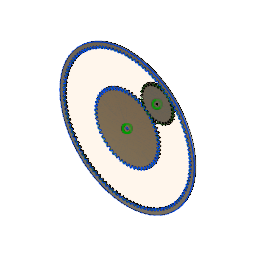
cncgearv3 (Autodesk Fusion 360 design; units mm, degrees)
description: Spur Gear; Module: 5.000000; Num Teeth: 56; Pressure Angle: 20.000000;
description: Spur Gear; Module: 5.000000; Num Teeth: 28; Pressure Angle: 20.000000;
description: Internal Gear; Module: 5.000000; Num Teeth: 112; Pressure Angle: 20.000000;
Autodesk Fusion 360 part; units mm, degrees
(part 1 of 4)
sketch "sketch 243" plane through (0, 0, 0) normal (0, 1, 0) x (1, 0, 0)
  spline S0 degree 3 poles (-118.3417, 63.013) (-119.0377, 63.2246) (-119.8918, 63.4524) (-120.912, 63.6705) knots 0 0 0 0 1 1 1 1
  arc A0 (-129.7827, 64.6689) -> (-131.4784, 61.1478) centre (0, 0) ccw
  spline S1 degree 3 poles (-125.167, 54.8349) (-124.3604, 54.1733) (-123.6498, 53.6475) (-123.0504, 53.2353) knots 0 0 0 0 1 1 1 1
  spline S2 degree 3 poles (-137.4981, 46.0424) (-134.792, 43.4861) (-132.4072, 41.6981) (-130.5195, 40.4758) knots 0 0 0 0 1 1 1 1
  spline S3 degree 3 poles (-130.5195, 40.4758) (-129.6439, 39.9087) (-128.8789, 39.4658) (-128.2371, 39.1233) knots 0 0 0 0 1 1 1 1
  spline S4 degree 3 poles (-129.3963, 35.0996) (-130.122, 35.1511) (-131.0054, 35.183) (-132.0485, 35.1687) knots 0 0 0 0 1 1 1 1
  arc A1 (-128.0426, 38.6549) -> (-128.2371, 39.1233) centre (-128.4255, 38.7705) ccw
  arc A2 (-136.2073, 49.7313) -> (-137.4981, 46.0424) centre (0, 0) ccw
  arc A3 (-129.3963, 35.0996) -> (-128.9824, 35.3927) centre (-129.3682, 35.4986) ccw
  spline S5 degree 3 poles (-141.7886, 30.358) (-138.8134, 28.1207) (-136.2434, 26.611) (-134.2307, 25.6078) knots 0 0 0 0 1 1 1 1
  arc A4 (-132.5126, 20.3911) -> (-132.1341, 20.7287) centre (-132.5293, 20.7907) ccw
  spline S6 degree 3 poles (-135.1558, 20.1628) (-137.3869, 19.8806) (-140.3113, 19.3045) (-143.8585, 18.1754) knots 0 0 0 0 1 1 1 1
  arc A5 (-133.4338, 9.1936) -> (-133.6242, 5.8041) centre (0, 0) ccw
  spline S7 degree 3 poles (-144.2961, 14.2918) (-141.0891, 12.4017) (-138.3662, 11.1893) (-136.2538, 10.4177) knots 0 0 0 0 1 1 1 1
  arc A6 (-116.2308, 66.1779) -> (-116.3162, 66.6779) centre (-116.5784, 66.3758) ccw
  arc A7 (-118.3417, 63.013) -> (-117.8729, 63.2067) centre (-118.2255, 63.3957) ccw
  arc A8 (-144.989, 1.9541) -> (-144.989, -1.9541) centre (0, 0) ccw
  spline S8 degree 3 poles (-144.989, -1.9541) (-141.5905, -3.4732) (-138.749, -4.3732) (-136.5635, -4.9034) knots 0 0 0 0 1 1 1 1
  spline S9 degree 3 poles (-136.5635, 4.9034) (-138.749, 4.3732) (-141.5905, 3.4732) (-144.989, 1.9541) knots 0 0 0 0 1 1 1 1
  arc A9 (-133.4338, 9.1936) -> (-133.7277, 9.607) centre (-133.8329, 9.2211) ccw
  arc A10 (-122.9095, 52.7481) -> (-124.2087, 49.6116) centre (0, 0) ccw
  spline S10 degree 3 poles (-110.5424, 75.8668) (-111.2103, 76.1551) (-112.0336, 76.477) (-113.0228, 76.808) knots 0 0 0 0 1 1 1 1
  spline S11 degree 3 poles (-118.2404, 68.5043) (-117.5129, 67.7566) (-116.8657, 67.1545) (-116.3162, 66.6779) knots 0 0 0 0 1 1 1 1
  spline S12 degree 3 poles (-120.912, 63.6705) (-123.1111, 64.141) (-126.0616, 64.5631) (-129.7827, 64.6689) knots 0 0 0 0 1 1 1 1
  arc A11 (-122.9095, 52.7481) -> (-123.0504, 53.2353) centre (-123.2771, 52.9058) ccw
  spline S13 degree 3 poles (-127.2805, 49.7323) (-129.5185, 49.9537) (-132.4978, 50.0427) (-136.2073, 49.7313) knots 0 0 0 0 1 1 1 1
  arc A12 (-128.0426, 38.6549) -> (-128.9824, 35.3927) centre (0, 0) ccw
  spline S14 degree 3 poles (-131.4784, 61.1478) (-129.0756, 58.3046) (-126.906, 56.2608) (-125.167, 54.8349) knots 0 0 0 0 1 1 1 1
  arc A13 (-140.919, 34.1682) -> (-141.7886, 30.358) centre (0, 0) ccw
  arc A14 (-131.5655, 24.0756) -> (-131.8112, 24.5193) centre (-131.9589, 24.1476) ccw
  spline S15 degree 3 poles (-134.2307, 25.6078) (-133.2971, 25.1423) (-132.4873, 24.7878) (-131.8112, 24.5193) knots 0 0 0 0 1 1 1 1
  arc A15 (-131.5655, 24.0756) -> (-132.1341, 20.7287) centre (0, 0) ccw
  spline S16 degree 3 poles (-132.5126, 20.3911) (-133.2394, 20.361) (-134.1209, 20.2939) (-135.1558, 20.1628) knots 0 0 0 0 1 1 1 1
  arc A16 (-143.8585, 18.1754) -> (-144.2961, 14.2918) centre (0, 0) ccw
  arc A17 (-124.6528, 49.3667) -> (-124.2087, 49.6116) centre (-124.5801, 49.76) ccw
  arc A18 (-116.2308, 66.1779) -> (-117.8729, 63.2067) centre (0, 0) ccw
  spline S17 degree 3 poles (-132.0485, 35.1687) (-134.2971, 35.1381) (-137.2676, 34.893) (-140.919, 34.1682) knots 0 0 0 0 1 1 1 1
  spline S18 degree 3 poles (-136.2538, 10.4177) (-135.274, 10.0596) (-134.4296, 9.798) (-133.7277, 9.607) knots 0 0 0 0 1 1 1 1
  spline S19 degree 3 poles (-133.9625, 5.4262) (-134.6814, 5.3149) (-135.5497, 5.1495) (-136.5635, 4.9034) knots 0 0 0 0 1 1 1 1
  arc A19 (-133.7277, -9.607) -> (-133.4338, -9.1936) centre (-133.8329, -9.2211) ccw
  arc A20 (-133.6242, -5.8041) -> (-133.9625, -5.4262) centre (-134.0238, -5.8214) ccw
  arc A21 (-133.6242, -5.8041) -> (-133.4338, -9.1936) centre (0, 0) ccw
  spline S20 degree 3 poles (-123.8053, 75.4842) (-121.7359, 72.3898) (-119.8088, 70.116) (-118.2404, 68.5043) knots 0 0 0 0 1 1 1 1
  spline S21 degree 3 poles (-124.6528, 49.3667) (-125.3681, 49.4991) (-126.2424, 49.6298) (-127.2805, 49.7323) knots 0 0 0 0 1 1 1 1
  arc A22 (-133.9625, 5.4262) -> (-133.6242, 5.8041) centre (-134.0238, 5.8214) ccw
  arc A23 (-121.726, 78.7934) -> (-123.8053, 75.4842) centre (0, 0) ccw
  spline S22 degree 3 poles (-113.0228, 76.808) (-115.1555, 77.5218) (-118.0402, 78.2715) (-121.726, 78.7934) knots 0 0 0 0 1 1 1 1
  spline S23 degree 3 poles (-136.2538, -10.4177) (-138.3662, -11.1893) (-141.0891, -12.4017) (-144.2961, -14.2918) knots 0 0 0 0 1 1 1 1
  spline S24 degree 3 poles (-135.1558, -20.1628) (-134.1209, -20.2939) (-133.2394, -20.361) (-132.5126, -20.3911) knots 0 0 0 0 1 1 1 1
  spline S25 degree 3 poles (-134.2307, -25.6078) (-136.2434, -26.611) (-138.8134, -28.1207) (-141.7886, -30.358) knots 0 0 0 0 1 1 1 1
  spline S26 degree 3 poles (-128.2371, -39.1233) (-128.8789, -39.4658) (-129.6439, -39.9087) (-130.5195, -40.4758) knots 0 0 0 0 1 1 1 1
  arc A24 (-110.0549, -76.0068) -> (-110.5424, -75.8668) centre (-110.384, -76.2341) ccw
  arc A25 (-128.2371, -39.1233) -> (-128.0426, -38.6549) centre (-128.4255, -38.7705) ccw
  spline S27 degree 3 poles (-108.1193, -79.2819) (-108.6119, -79.8171) (-109.1877, -80.4878) (-109.8269, -81.3123) knots 0 0 0 0 1 1 1 1
  arc A26 (-110.0549, -76.0068) -> (-108.0904, -78.7755) centre (0, 0) ccw
  arc A27 (-128.9824, -35.3927) -> (-129.3963, -35.0996) centre (-129.3682, -35.4986) ccw
  spline S28 degree 3 poles (-136.2073, -49.7313) (-132.4978, -50.0427) (-129.5185, -49.9537) (-127.2805, -49.7323) knots 0 0 0 0 1 1 1 1
  spline S29 degree 3 poles (-103.7124, -88.9796) (-102.7664, -88.5399) (-101.9843, -88.1278) (-101.3529, -87.7666) knots 0 0 0 0 1 1 1 1
  spline S30 degree 3 poles (-109.8269, -81.3123) (-111.205, -83.0895) (-112.8654, -85.5648) (-114.5753, -88.8714) knots 0 0 0 0 1 1 1 1
  spline S31 degree 3 poles (-118.2404, -68.5043) (-119.8088, -70.116) (-121.7359, -72.3898) (-123.8053, -75.4842) knots 0 0 0 0 1 1 1 1
  spline S32 degree 3 poles (-112.1386, -91.9269) (-108.5344, -90.9957) (-105.7517, -89.9277) (-103.7124, -88.9796) knots 0 0 0 0 1 1 1 1
  arc A28 (-114.5753, -88.8714) -> (-112.1386, -91.9269) centre (0, 0) ccw
  spline S33 degree 3 poles (-129.7827, -64.6689) (-126.0616, -64.5631) (-123.1111, -64.141) (-120.912, -63.6705) knots 0 0 0 0 1 1 1 1
  arc A29 (-100.8528, -87.8511) -> (-101.3529, -87.7666) centre (-101.1544, -88.1139) ccw
  arc A30 (-132.1341, -20.7287) -> (-131.5655, -24.0756) centre (0, 0) ccw
  arc A31 (-131.8112, -24.5193) -> (-131.5655, -24.0756) centre (-131.9589, -24.1476) ccw
  arc A32 (-123.0504, -53.2353) -> (-122.9095, -52.7481) centre (-123.2771, -52.9058) ccw
  spline S34 degree 3 poles (-125.167, -54.8349) (-126.906, -56.2608) (-129.0756, -58.3046) (-131.4784, -61.1478) knots 0 0 0 0 1 1 1 1
  arc A33 (-131.4784, -61.1478) -> (-129.7827, -64.6689) centre (0, 0) ccw
  arc A34 (-116.3162, -66.6779) -> (-116.2308, -66.1779) centre (-116.5784, -66.3758) ccw
  spline S35 degree 3 poles (-136.5635, -4.9034) (-135.5497, -5.1495) (-134.6814, -5.3149) (-133.9625, -5.4262) knots 0 0 0 0 1 1 1 1
  spline S36 degree 3 poles (-130.5195, -40.4758) (-132.4072, -41.6981) (-134.792, -43.4861) (-137.4981, -46.0424) knots 0 0 0 0 1 1 1 1
  arc A35 (-117.8729, -63.2067) -> (-118.3417, -63.013) centre (-118.2255, -63.3957) ccw
  arc A36 (-128.9824, -35.3927) -> (-128.0426, -38.6549) centre (0, 0) ccw
  spline S37 degree 3 poles (-116.3162, -66.6779) (-116.8657, -67.1545) (-117.5129, -67.7566) (-118.2404, -68.5043) knots 0 0 0 0 1 1 1 1
  arc A37 (-117.8729, -63.2067) -> (-116.2308, -66.1779) centre (0, 0) ccw
  spline S38 degree 3 poles (-131.8112, -24.5193) (-132.4873, -24.7878) (-133.2971, -25.1423) (-134.2307, -25.6078) knots 0 0 0 0 1 1 1 1
  arc A38 (-137.4981, -46.0424) -> (-136.2073, -49.7313) centre (0, 0) ccw
  spline S39 degree 3 poles (-132.0485, -35.1687) (-131.0054, -35.183) (-130.122, -35.1511) (-129.3963, -35.0996) knots 0 0 0 0 1 1 1 1
  spline S40 degree 3 poles (-143.8585, -18.1754) (-140.3113, -19.3045) (-137.3869, -19.8806) (-135.1558, -20.1628) knots 0 0 0 0 1 1 1 1
  spline S41 degree 3 poles (-140.919, -34.1682) (-137.2676, -34.893) (-134.2971, -35.1381) (-132.0485, -35.1687) knots 0 0 0 0 1 1 1 1
  arc A39 (-141.7886, -30.358) -> (-140.919, -34.1682) centre (0, 0) ccw
  arc A40 (-124.2087, -49.6116) -> (-122.9095, -52.7481) centre (0, 0) ccw
  arc A41 (-124.2087, -49.6116) -> (-124.6528, -49.3667) centre (-124.5801, -49.76) ccw
  spline S42 degree 3 poles (-123.0504, -53.2353) (-123.6498, -53.6475) (-124.3604, -54.1733) (-125.167, -54.8349) knots 0 0 0 0 1 1 1 1
  spline S43 degree 3 poles (-120.912, -63.6705) (-119.8918, -63.4524) (-119.0377, -63.2246) (-118.3417, -63.013) knots 0 0 0 0 1 1 1 1
  spline S44 degree 3 poles (-121.726, -78.7934) (-118.0402, -78.2715) (-115.1555, -77.5218) (-113.0228, -76.808) knots 0 0 0 0 1 1 1 1
  arc A42 (-123.8053, -75.4842) -> (-121.726, -78.7934) centre (0, 0) ccw
  spline S45 degree 3 poles (-113.0228, -76.808) (-112.0336, -76.477) (-111.2103, -76.1551) (-110.5424, -75.8668) knots 0 0 0 0 1 1 1 1
  arc A43 (-144.2961, -14.2918) -> (-143.8585, -18.1754) centre (0, 0) ccw
  spline S46 degree 3 poles (-127.2805, -49.7323) (-126.2424, -49.6298) (-125.3681, -49.4991) (-124.6528, -49.3667) knots 0 0 0 0 1 1 1 1
  arc A44 (-108.1193, -79.2819) -> (-108.0904, -78.7755) centre (-108.4136, -79.0111) ccw
  arc A45 (-132.1341, -20.7287) -> (-132.5126, -20.3911) centre (-132.5293, -20.7907) ccw
  spline S47 degree 3 poles (-133.7277, -9.607) (-134.4296, -9.798) (-135.274, -10.0596) (-136.2538, -10.4177) knots 0 0 0 0 1 1 1 1
  spline S48 degree 3 poles (-75.8668, -110.5424) (-76.1551, -111.2103) (-76.477, -112.0336) (-76.808, -113.0228) knots 0 0 0 0 1 1 1 1
  spline S49 degree 3 poles (-93.0977, -100.0322) (-92.2069, -99.4894) (-91.4759, -98.9923) (-90.8889, -98.5627) knots 0 0 0 0 1 1 1 1
  spline S50 degree 3 poles (-87.7666, -101.3529) (-88.1278, -101.9843) (-88.5399, -102.7664) (-88.9796, -103.7124) knots 0 0 0 0 1 1 1 1
  arc A46 (-78.7755, -108.0904) -> (-79.2819, -108.1193) centre (-79.0111, -108.4136) ccw
  arc A47 (-75.8668, -110.5424) -> (-76.0068, -110.0549) centre (-76.2341, -110.384) ccw
  spline S51 degree 3 poles (-76.808, -113.0228) (-77.5218, -115.1555) (-78.2715, -118.0402) (-78.7934, -121.726) knots 0 0 0 0 1 1 1 1
  arc A48 (-90.3825, -98.5907) -> (-90.8889, -98.5627) centre (-90.6528, -98.8855) ccw
  arc A49 (-78.7934, -121.726) -> (-75.4842, -123.8053) centre (0, 0) ccw
  spline S52 degree 3 poles (-75.4842, -123.8053) (-72.3898, -121.7359) (-70.116, -119.8088) (-68.5043, -118.2404) knots 0 0 0 0 1 1 1 1
  arc A50 (-66.1779, -116.2308) -> (-63.2067, -117.8729) centre (0, 0) ccw
  arc A51 (-63.013, -118.3417) -> (-63.2067, -117.8729) centre (-63.3957, -118.2255) ccw
  spline S53 degree 3 poles (-100.0322, -93.0977) (-101.2027, -95.018) (-102.5755, -97.6637) (-103.9044, -101.1409) knots 0 0 0 0 1 1 1 1
  spline S54 degree 3 poles (-88.9796, -103.7124) (-89.9277, -105.7517) (-90.9957, -108.5344) (-91.9269, -112.1386) knots 0 0 0 0 1 1 1 1
  arc A52 (-100.8528, -87.8511) -> (-98.5907, -90.3825) centre (0, 0) ccw
  spline S55 degree 3 poles (-81.3123, -109.8269) (-80.4878, -109.1877) (-79.8171, -108.6119) (-79.2819, -108.1193) knots 0 0 0 0 1 1 1 1
  spline S56 degree 3 poles (-88.8714, -114.5753) (-85.5648, -112.8654) (-83.0895, -111.205) (-81.3123, -109.8269) knots 0 0 0 0 1 1 1 1
  arc A53 (-91.9269, -112.1386) -> (-88.8714, -114.5753) centre (0, 0) ccw
  arc A54 (-90.3825, -98.5907) -> (-87.8511, -100.8528) centre (0, 0) ccw
  arc A55 (-66.1779, -116.2308) -> (-66.6779, -116.3162) centre (-66.3758, -116.5784) ccw
  spline S57 degree 3 poles (-101.1409, -103.9044) (-97.6637, -102.5755) (-95.018, -101.2027) (-93.0977, -100.0322) knots 0 0 0 0 1 1 1 1
  arc A56 (-78.7755, -108.0904) -> (-76.0068, -110.0549) centre (0, 0) ccw
  spline S58 degree 3 poles (-68.5043, -118.2404) (-67.7566, -117.5129) (-67.1545, -116.8657) (-66.6779, -116.3162) knots 0 0 0 0 1 1 1 1
  arc A57 (-103.9044, -101.1409) -> (-101.1409, -103.9044) centre (0, 0) ccw
  spline S59 degree 3 poles (-63.013, -118.3417) (-63.2246, -119.0377) (-63.4524, -119.8918) (-63.6705, -120.912) knots 0 0 0 0 1 1 1 1
  arc A58 (-87.7666, -101.3529) -> (-87.8511, -100.8528) centre (-88.1139, -101.1544) ccw
  spline S60 degree 3 poles (-54.8349, -125.167) (-54.1733, -124.3604) (-53.6475, -123.6498) (-53.2353, -123.0504) knots 0 0 0 0 1 1 1 1
  spline S61 degree 3 poles (-98.5627, -90.8889) (-98.9923, -91.4759) (-99.4894, -92.2069) (-100.0322, -93.0977) knots 0 0 0 0 1 1 1 1
  arc A59 (-98.5627, -90.8889) -> (-98.5907, -90.3825) centre (-98.8855, -90.6528) ccw
  spline S62 degree 3 poles (-63.6705, -120.912) (-64.141, -123.1111) (-64.5631, -126.0616) (-64.6689, -129.7827) knots 0 0 0 0 1 1 1 1
  spline S63 degree 3 poles (-61.1478, -131.4784) (-58.3046, -129.0756) (-56.2608, -126.906) (-54.8349, -125.167) knots 0 0 0 0 1 1 1 1
  arc A60 (-88.8714, 114.5753) -> (-91.9269, 112.1386) centre (0, 0) ccw
  spline S64 degree 3 poles (-88.9796, 103.7124) (-88.5399, 102.7664) (-88.1278, 101.9843) (-87.7666, 101.3529) knots 0 0 0 0 1 1 1 1
  arc A61 (-87.8511, 100.8528) -> (-87.7666, 101.3529) centre (-88.1139, 101.1544) ccw
  spline S65 degree 3 poles (-90.8889, 98.5627) (-91.4759, 98.9923) (-92.2069, 99.4894) (-93.0977, 100.0322) knots 0 0 0 0 1 1 1 1
  arc A62 (-90.8889, 98.5627) -> (-90.3825, 98.5907) centre (-90.6528, 98.8855) ccw
  spline S66 degree 3 poles (-93.0977, 100.0322) (-95.018, 101.2027) (-97.6637, 102.5755) (-101.1409, 103.9044) knots 0 0 0 0 1 1 1 1
  arc A63 (-64.6689, -129.7827) -> (-61.1478, -131.4784) centre (0, 0) ccw
  spline S67 degree 3 poles (-91.9269, 112.1386) (-90.9957, 108.5344) (-89.9277, 105.7517) (-88.9796, 103.7124) knots 0 0 0 0 1 1 1 1
  spline S68 degree 3 poles (-103.9044, 101.1409) (-102.5755, 97.6637) (-101.2027, 95.018) (-100.0322, 93.0977) knots 0 0 0 0 1 1 1 1
  spline S69 degree 3 poles (-81.3123, 109.8269) (-83.0895, 111.205) (-85.5648, 112.8654) (-88.8714, 114.5753) knots 0 0 0 0 1 1 1 1
  arc A64 (-87.8511, 100.8528) -> (-90.3825, 98.5907) centre (0, 0) ccw
  arc A65 (-98.5907, 90.3825) -> (-100.8528, 87.8511) centre (0, 0) ccw
  arc A66 (-108.0904, 78.7755) -> (-108.1193, 79.2819) centre (-108.4136, 79.0111) ccw
  arc A67 (-110.5424, 75.8668) -> (-110.0549, 76.0068) centre (-110.384, 76.2341) ccw
  arc A68 (-108.0904, 78.7755) -> (-110.0549, 76.0068) centre (0, 0) ccw
  arc A69 (24.5193, -131.8112) -> (24.0756, -131.5655) centre (24.1476, -131.9589) ccw
  arc A70 (14.2918, -144.2961) -> (18.1754, -143.8585) centre (0, 0) ccw
  spline S70 degree 3 poles (20.1628, -135.1558) (20.2939, -134.1209) (20.361, -133.2394) (20.3911, -132.5126) knots 0 0 0 0 1 1 1 1
  spline S71 degree 3 poles (18.1754, -143.8585) (19.3045, -140.3113) (19.8806, -137.3869) (20.1628, -135.1558) knots 0 0 0 0 1 1 1 1
  arc A71 (20.7287, -132.1341) -> (20.3911, -132.5126) centre (20.7907, -132.5293) ccw
  spline S72 degree 3 poles (25.6078, -134.2307) (26.611, -136.2434) (28.1207, -138.8134) (30.358, -141.7886) knots 0 0 0 0 1 1 1 1
  spline S73 degree 3 poles (34.1682, -140.919) (34.893, -137.2676) (35.1381, -134.2971) (35.1687, -132.0485) knots 0 0 0 0 1 1 1 1
  arc A72 (35.3927, -128.9824) -> (35.0996, -129.3963) centre (35.4986, -129.3682) ccw
  arc A73 (35.3927, -128.9824) -> (38.6549, -128.0426) centre (0, 0) ccw
  spline S74 degree 3 poles (-103.7124, 88.9796) (-105.7517, 89.9277) (-108.5344, 90.9957) (-112.1386, 91.9269) knots 0 0 0 0 1 1 1 1
  spline S75 degree 3 poles (-100.0322, 93.0977) (-99.4894, 92.2069) (-98.9923, 91.4759) (-98.5627, 90.8889) knots 0 0 0 0 1 1 1 1
  spline S76 degree 3 poles (-109.8269, 81.3123) (-109.1877, 80.4878) (-108.6119, 79.8171) (-108.1193, 79.2819) knots 0 0 0 0 1 1 1 1
  spline S77 degree 3 poles (40.4758, -130.5195) (41.6981, -132.4072) (43.4861, -134.792) (46.0424, -137.4981) knots 0 0 0 0 1 1 1 1
  spline S78 degree 3 poles (39.1233, -128.2371) (39.4658, -128.8789) (39.9087, -129.6439) (40.4758, -130.5195) knots 0 0 0 0 1 1 1 1
  arc A74 (53.2353, -123.0504) -> (52.7481, -122.9095) centre (52.9058, -123.2771) ccw
  arc A75 (49.6116, -124.2087) -> (49.3667, -124.6528) centre (49.76, -124.5801) ccw
  spline S79 degree 3 poles (-114.5753, 88.8714) (-112.8654, 85.5648) (-111.205, 83.0895) (-109.8269, 81.3123) knots 0 0 0 0 1 1 1 1
  spline S80 degree 3 poles (24.5193, -131.8112) (24.7878, -132.4873) (25.1423, -133.2971) (25.6078, -134.2307) knots 0 0 0 0 1 1 1 1
  spline S81 degree 3 poles (35.1687, -132.0485) (35.183, -131.0054) (35.1511, -130.122) (35.0996, -129.3963) knots 0 0 0 0 1 1 1 1
  arc A76 (-101.3529, 87.7666) -> (-100.8528, 87.8511) centre (-101.1544, 88.1139) ccw
  arc A77 (20.7287, -132.1341) -> (24.0756, -131.5655) centre (0, 0) ccw
  arc A78 (30.358, -141.7886) -> (34.1682, -140.919) centre (0, 0) ccw
  arc A79 (39.1233, -128.2371) -> (38.6549, -128.0426) centre (38.7705, -128.4255) ccw
  arc A80 (46.0424, -137.4981) -> (49.7313, -136.2073) centre (0, 0) ccw
  spline S82 degree 3 poles (53.2353, -123.0504) (53.6475, -123.6498) (54.1733, -124.3604) (54.8349, -125.167) knots 0 0 0 0 1 1 1 1
  spline S83 degree 3 poles (49.7313, -136.2073) (50.0427, -132.4978) (49.9537, -129.5185) (49.7323, -127.2805) knots 0 0 0 0 1 1 1 1
  arc A81 (-98.5907, 90.3825) -> (-98.5627, 90.8889) centre (-98.8855, 90.6528) ccw
  spline S84 degree 3 poles (-101.3529, 87.7666) (-101.9843, 88.1278) (-102.7664, 88.5399) (-103.7124, 88.9796) knots 0 0 0 0 1 1 1 1
  arc A82 (-112.1386, 91.9269) -> (-114.5753, 88.8714) centre (0, 0) ccw
  arc A83 (-101.1409, 103.9044) -> (-103.9044, 101.1409) centre (0, 0) ccw
  spline S85 degree 3 poles (137.4981, -46.0424) (134.792, -43.4861) (132.4072, -41.6981) (130.5195, -40.4758) knots 0 0 0 0 1 1 1 1
  spline S86 degree 3 poles (90.8889, -98.5627) (91.4759, -98.9923) (92.2069, -99.4894) (93.0977, -100.0322) knots 0 0 0 0 1 1 1 1
  arc A84 (88.8714, -114.5753) -> (91.9269, -112.1386) centre (0, 0) ccw
  arc A85 (128.0426, -38.6549) -> (128.9824, -35.3927) centre (0, 0) ccw
  arc A86 (49.6116, -124.2087) -> (52.7481, -122.9095) centre (0, 0) ccw
  spline S87 degree 3 poles (101.3529, -87.7666) (101.9843, -88.1278) (102.7664, -88.5399) (103.7124, -88.9796) knots 0 0 0 0 1 1 1 1
  arc A87 (108.0904, -78.7755) -> (110.0549, -76.0068) centre (0, 0) ccw
  arc A88 (116.2308, -66.1779) -> (116.3162, -66.6779) centre (116.5784, -66.3758) ccw
  spline S88 degree 3 poles (88.9796, -103.7124) (88.5399, -102.7664) (88.1278, -101.9843) (87.7666, -101.3529) knots 0 0 0 0 1 1 1 1
  arc A89 (110.5424, -75.8668) -> (110.0549, -76.0068) centre (110.384, -76.2341) ccw
  arc A90 (63.2067, -117.8729) -> (66.1779, -116.2308) centre (0, 0) ccw
  spline S89 degree 3 poles (103.9044, -101.1409) (102.5755, -97.6637) (101.2027, -95.018) (100.0322, -93.0977) knots 0 0 0 0 1 1 1 1
  spline S90 degree 3 poles (66.6779, -116.3162) (67.1545, -116.8657) (67.7566, -117.5129) (68.5043, -118.2404) knots 0 0 0 0 1 1 1 1
  arc A91 (122.9095, -52.7481) -> (123.0504, -53.2353) centre (123.2771, -52.9058) ccw
  spline S91 degree 3 poles (78.7934, -121.726) (78.2715, -118.0402) (77.5218, -115.1555) (76.808, -113.0228) knots 0 0 0 0 1 1 1 1
  arc A92 (112.1386, -91.9269) -> (114.5753, -88.8714) centre (0, 0) ccw
  arc A93 (121.726, -78.7934) -> (123.8053, -75.4842) centre (0, 0) ccw
  spline S92 degree 3 poles (76.808, -113.0228) (76.477, -112.0336) (76.1551, -111.2103) (75.8668, -110.5424) knots 0 0 0 0 1 1 1 1
  arc A94 (75.4842, -123.8053) -> (78.7934, -121.726) centre (0, 0) ccw
  arc A95 (61.1478, -131.4784) -> (64.6689, -129.7827) centre (0, 0) ccw
  spline S93 degree 3 poles (68.5043, -118.2404) (70.116, -119.8088) (72.3898, -121.7359) (75.4842, -123.8053) knots 0 0 0 0 1 1 1 1
  arc A96 (87.8511, -100.8528) -> (87.7666, -101.3529) centre (88.1139, -101.1544) ccw
  arc A97 (76.0068, -110.0549) -> (75.8668, -110.5424) centre (76.2341, -110.384) ccw
  spline S94 degree 3 poles (110.5424, -75.8668) (111.2103, -76.1551) (112.0336, -76.477) (113.0228, -76.808) knots 0 0 0 0 1 1 1 1
  spline S95 degree 3 poles (100.0322, -93.0977) (99.4894, -92.2069) (98.9923, -91.4759) (98.5627, -90.8889) knots 0 0 0 0 1 1 1 1
  arc A98 (101.3529, -87.7666) -> (100.8528, -87.8511) centre (101.1544, -88.1139) ccw
  arc A99 (101.1409, -103.9044) -> (103.9044, -101.1409) centre (0, 0) ccw
  spline S96 degree 3 poles (109.8269, -81.3123) (109.1877, -80.4878) (108.6119, -79.8171) (108.1193, -79.2819) knots 0 0 0 0 1 1 1 1
  spline S97 degree 3 poles (113.0228, -76.808) (115.1555, -77.5218) (118.0402, -78.2715) (121.726, -78.7934) knots 0 0 0 0 1 1 1 1
  spline S98 degree 3 poles (125.167, -54.8349) (124.3604, -54.1733) (123.6498, -53.6475) (123.0504, -53.2353) knots 0 0 0 0 1 1 1 1
  arc A100 (63.2067, -117.8729) -> (63.013, -118.3417) centre (63.3957, -118.2255) ccw
  arc A101 (122.9095, -52.7481) -> (124.2087, -49.6116) centre (0, 0) ccw
  spline S99 degree 3 poles (131.4784, -61.1478) (129.0756, -58.3046) (126.906, -56.2608) (125.167, -54.8349) knots 0 0 0 0 1 1 1 1
  arc A102 (87.8511, -100.8528) -> (90.3825, -98.5907) centre (0, 0) ccw
  arc A103 (90.8889, -98.5627) -> (90.3825, -98.5907) centre (90.6528, -98.8855) ccw
  spline S100 degree 3 poles (118.2404, -68.5043) (117.5129, -67.7566) (116.8657, -67.1545) (116.3162, -66.6779) knots 0 0 0 0 1 1 1 1
  spline S101 degree 3 poles (91.9269, -112.1386) (90.9957, -108.5344) (89.9277, -105.7517) (88.9796, -103.7124) knots 0 0 0 0 1 1 1 1
  arc A104 (116.2308, -66.1779) -> (117.8729, -63.2067) centre (0, 0) ccw
  spline S102 degree 3 poles (120.912, -63.6705) (123.1111, -64.141) (126.0616, -64.5631) (129.7827, -64.6689) knots 0 0 0 0 1 1 1 1
  spline S103 degree 3 poles (118.3417, -63.013) (119.0377, -63.2246) (119.8918, -63.4524) (120.912, -63.6705) knots 0 0 0 0 1 1 1 1
  arc A105 (98.5907, -90.3825) -> (100.8528, -87.8511) centre (0, 0) ccw
  arc A106 (66.6779, -116.3162) -> (66.1779, -116.2308) centre (66.3758, -116.5784) ccw
  spline S104 degree 3 poles (123.8053, -75.4842) (121.7359, -72.3898) (119.8088, -70.116) (118.2404, -68.5043) knots 0 0 0 0 1 1 1 1
  spline S105 degree 3 poles (93.0977, -100.0322) (95.018, -101.2027) (97.6637, -102.5755) (101.1409, -103.9044) knots 0 0 0 0 1 1 1 1
  arc A107 (129.7827, -64.6689) -> (131.4784, -61.1478) centre (0, 0) ccw
  arc A108 (79.2819, -108.1193) -> (78.7755, -108.0904) centre (79.0111, -108.4136) ccw
  spline S106 degree 3 poles (114.5753, -88.8714) (112.8654, -85.5648) (111.205, -83.0895) (109.8269, -81.3123) knots 0 0 0 0 1 1 1 1
  spline S107 degree 3 poles (63.6705, -120.912) (63.4524, -119.8918) (63.2246, -119.0377) (63.013, -118.3417) knots 0 0 0 0 1 1 1 1
  arc A109 (98.5907, -90.3825) -> (98.5627, -90.8889) centre (98.8855, -90.6528) ccw
  spline S108 degree 3 poles (124.6528, -49.3667) (125.3681, -49.4991) (126.2424, -49.6298) (127.2805, -49.7323) knots 0 0 0 0 1 1 1 1
  spline S109 degree 3 poles (103.7124, -88.9796) (105.7517, -89.9277) (108.5344, -90.9957) (112.1386, -91.9269) knots 0 0 0 0 1 1 1 1
  spline S110 degree 3 poles (64.6689, -129.7827) (64.5631, -126.0616) (64.141, -123.1111) (63.6705, -120.912) knots 0 0 0 0 1 1 1 1
  spline S111 degree 3 poles (81.3123, -109.8269) (83.0895, -111.205) (85.5648, -112.8654) (88.8714, -114.5753) knots 0 0 0 0 1 1 1 1
  arc A110 (124.6528, -49.3667) -> (124.2087, -49.6116) centre (124.5801, -49.76) ccw
  arc A111 (136.2073, -49.7313) -> (137.4981, -46.0424) centre (0, 0) ccw
  spline S112 degree 3 poles (127.2805, -49.7323) (129.5185, -49.9537) (132.4978, -50.0427) (136.2073, -49.7313) knots 0 0 0 0 1 1 1 1
  arc A112 (128.0426, -38.6549) -> (128.2371, -39.1233) centre (128.4255, -38.7705) ccw
  arc A113 (76.0068, -110.0549) -> (78.7755, -108.0904) centre (0, 0) ccw
  spline S113 degree 3 poles (130.5195, -40.4758) (129.6439, -39.9087) (128.8789, -39.4658) (128.2371, -39.1233) knots 0 0 0 0 1 1 1 1
  spline S114 degree 3 poles (49.7323, -127.2805) (49.6298, -126.2424) (49.4991, -125.3681) (49.3667, -124.6528) knots 0 0 0 0 1 1 1 1
  spline S115 degree 3 poles (54.8349, -125.167) (56.2608, -126.906) (58.3046, -129.0756) (61.1478, -131.4784) knots 0 0 0 0 1 1 1 1
  spline S116 degree 3 poles (79.2819, -108.1193) (79.8171, -108.6119) (80.4878, -109.1877) (81.3123, -109.8269) knots 0 0 0 0 1 1 1 1
  arc A114 (108.0904, -78.7755) -> (108.1193, -79.2819) centre (108.4136, -79.0111) ccw
  arc A115 (118.3417, -63.013) -> (117.8729, -63.2067) centre (118.2255, -63.3957) ccw
  spline S117 degree 3 poles (132.0485, -35.1687) (134.2971, -35.1381) (137.2676, -34.893) (140.919, -34.1682) knots 0 0 0 0 1 1 1 1
  spline S118 degree 3 poles (-49.7323, -127.2805) (-49.9537, -129.5185) (-50.0427, -132.4978) (-49.7313, -136.2073) knots 0 0 0 0 1 1 1 1
  spline S119 degree 3 poles (-40.4758, -130.5195) (-39.9087, -129.6439) (-39.4658, -128.8789) (-39.1233, -128.2371) knots 0 0 0 0 1 1 1 1
  arc A116 (140.919, -34.1682) -> (141.7886, -30.358) centre (0, 0) ccw
  arc A117 (133.4338, -9.1936) -> (133.7277, -9.607) centre (133.8329, -9.2211) ccw
  arc A118 (132.5126, -20.3911) -> (132.1341, -20.7287) centre (132.5293, -20.7907) ccw
  arc A119 (131.5655, -24.0756) -> (132.1341, -20.7287) centre (0, 0) ccw
  arc A120 (143.8585, -18.1754) -> (144.2961, -14.2918) centre (0, 0) ccw
  arc A121 (-52.7481, -122.9095) -> (-49.6116, -124.2087) centre (0, 0) ccw
  arc A122 (-49.3667, -124.6528) -> (-49.6116, -124.2087) centre (-49.76, -124.5801) ccw
  spline S120 degree 3 poles (-49.3667, -124.6528) (-49.4991, -125.3681) (-49.6298, -126.2424) (-49.7323, -127.2805) knots 0 0 0 0 1 1 1 1
  spline S121 degree 3 poles (-46.0424, -137.4981) (-43.4861, -134.792) (-41.6981, -132.4072) (-40.4758, -130.5195) knots 0 0 0 0 1 1 1 1
  arc A123 (-38.6549, -128.0426) -> (-39.1233, -128.2371) centre (-38.7705, -128.4255) ccw
  arc A124 (-38.6549, -128.0426) -> (-35.3927, -128.9824) centre (0, 0) ccw
  arc A125 (133.4338, -9.1936) -> (133.6242, -5.8041) centre (0, 0) ccw
  arc A126 (-35.0996, -129.3963) -> (-35.3927, -128.9824) centre (-35.4986, -129.3682) ccw
  arc A127 (129.3963, -35.0996) -> (128.9824, -35.3927) centre (129.3682, -35.4986) ccw
  arc A128 (-34.1682, -140.919) -> (-30.358, -141.7886) centre (0, 0) ccw
  spline S122 degree 3 poles (-35.0996, -129.3963) (-35.1511, -130.122) (-35.183, -131.0054) (-35.1687, -132.0485) knots 0 0 0 0 1 1 1 1
  spline S123 degree 3 poles (144.2961, -14.2918) (141.0891, -12.4017) (138.3662, -11.1893) (136.2538, -10.4177) knots 0 0 0 0 1 1 1 1
  spline S124 degree 3 poles (132.5126, -20.3911) (133.2394, -20.361) (134.1209, -20.2939) (135.1558, -20.1628) knots 0 0 0 0 1 1 1 1
  spline S125 degree 3 poles (135.1558, -20.1628) (137.3869, -19.8806) (140.3113, -19.3045) (143.8585, -18.1754) knots 0 0 0 0 1 1 1 1
  spline S126 degree 3 poles (129.3963, -35.0996) (130.122, -35.1511) (131.0054, -35.183) (132.0485, -35.1687) knots 0 0 0 0 1 1 1 1
  spline S127 degree 3 poles (134.2307, -25.6078) (133.2971, -25.1423) (132.4873, -24.7878) (131.8112, -24.5193) knots 0 0 0 0 1 1 1 1
  arc A129 (131.5655, -24.0756) -> (131.8112, -24.5193) centre (131.9589, -24.1476) ccw
  spline S128 degree 3 poles (141.7886, -30.358) (138.8134, -28.1207) (136.2434, -26.611) (134.2307, -25.6078) knots 0 0 0 0 1 1 1 1
  circle A130 centre (0, 0) radius 4
  spline S129 degree 3 poles (136.2538, -10.4177) (135.274, -10.0596) (134.4296, -9.798) (133.7277, -9.607) knots 0 0 0 0 1 1 1 1
  arc A131 (-52.7481, -122.9095) -> (-53.2353, -123.0504) centre (-52.9058, -123.2771) ccw
  arc A132 (-49.7313, -136.2073) -> (-46.0424, -137.4981) centre (0, 0) ccw
  spline S130 degree 3 poles (127.2805, 49.7323) (126.2424, 49.6298) (125.3681, 49.4991) (124.6528, 49.3667) knots 0 0 0 0 1 1 1 1
  arc A133 (-9.1936, -133.4338) -> (-5.8041, -133.6242) centre (0, 0) ccw
  arc A134 (-24.0756, -131.5655) -> (-24.5193, -131.8112) centre (-24.1476, -131.9589) ccw
  arc A135 (144.989, -1.9541) -> (144.989, 1.9541) centre (0, 0) ccw
  arc A136 (131.8112, 24.5193) -> (131.5655, 24.0756) centre (131.9589, 24.1476) ccw
  arc A137 (5.8041, -133.6242) -> (9.1936, -133.4338) centre (0, 0) ccw
  arc A138 (-18.1754, -143.8585) -> (-14.2918, -144.2961) centre (0, 0) ccw
  arc A139 (133.6242, 5.8041) -> (133.9625, 5.4262) centre (134.0238, 5.8214) ccw
  spline S131 degree 3 poles (134.2307, 25.6078) (136.2434, 26.611) (138.8134, 28.1207) (141.7886, 30.358) knots 0 0 0 0 1 1 1 1
  spline S132 degree 3 poles (-20.1628, -135.1558) (-19.8806, -137.3869) (-19.3045, -140.3113) (-18.1754, -143.8585) knots 0 0 0 0 1 1 1 1
  spline S133 degree 3 poles (136.5635, 4.9034) (135.5497, 5.1495) (134.6814, 5.3149) (133.9625, 5.4262) knots 0 0 0 0 1 1 1 1
  spline S134 degree 3 poles (136.2538, 10.4177) (138.3662, 11.1893) (141.0891, 12.4017) (144.2961, 14.2918) knots 0 0 0 0 1 1 1 1
  arc A140 (132.1341, 20.7287) -> (132.5126, 20.3911) centre (132.5293, 20.7907) ccw
  spline S135 degree 3 poles (133.7277, 9.607) (134.4296, 9.798) (135.274, 10.0596) (136.2538, 10.4177) knots 0 0 0 0 1 1 1 1
  arc A141 (141.7886, 30.358) -> (140.919, 34.1682) centre (0, 0) ccw
  spline S136 degree 3 poles (131.8112, 24.5193) (132.4873, 24.7878) (133.2971, 25.1423) (134.2307, 25.6078) knots 0 0 0 0 1 1 1 1
  spline S137 degree 3 poles (-30.358, -141.7886) (-28.1207, -138.8134) (-26.611, -136.2434) (-25.6078, -134.2307) knots 0 0 0 0 1 1 1 1
  spline S138 degree 3 poles (9.607, -133.7277) (9.798, -134.4296) (10.0596, -135.274) (10.4177, -136.2538) knots 0 0 0 0 1 1 1 1
  spline S139 degree 3 poles (144.989, 1.9541) (141.5905, 3.4732) (138.749, 4.3732) (136.5635, 4.9034) knots 0 0 0 0 1 1 1 1
  spline S140 degree 3 poles (133.9625, -5.4262) (134.6814, -5.3149) (135.5497, -5.1495) (136.5635, -4.9034) knots 0 0 0 0 1 1 1 1
  arc A142 (132.1341, 20.7287) -> (131.5655, 24.0756) centre (0, 0) ccw
  spline S141 degree 3 poles (136.5635, -4.9034) (138.749, -4.3732) (141.5905, -3.4732) (144.989, -1.9541) knots 0 0 0 0 1 1 1 1
  spline S142 degree 3 poles (140.919, 34.1682) (137.2676, 34.893) (134.2971, 35.1381) (132.0485, 35.1687) knots 0 0 0 0 1 1 1 1
  arc A143 (128.9824, 35.3927) -> (129.3963, 35.0996) centre (129.3682, 35.4986) ccw
  spline S143 degree 3 poles (135.1558, 20.1628) (134.1209, 20.2939) (133.2394, 20.361) (132.5126, 20.3911) knots 0 0 0 0 1 1 1 1
  spline S144 degree 3 poles (132.0485, 35.1687) (131.0054, 35.183) (130.122, 35.1511) (129.3963, 35.0996) knots 0 0 0 0 1 1 1 1
  spline S145 degree 3 poles (4.9034, -136.5635) (5.1495, -135.5497) (5.3149, -134.6814) (5.4262, -133.9625) knots 0 0 0 0 1 1 1 1
  spline S146 degree 3 poles (-20.3911, -132.5126) (-20.361, -133.2394) (-20.2939, -134.1209) (-20.1628, -135.1558) knots 0 0 0 0 1 1 1 1
  spline S147 degree 3 poles (128.2371, 39.1233) (128.8789, 39.4658) (129.6439, 39.9087) (130.5195, 40.4758) knots 0 0 0 0 1 1 1 1
  arc A144 (137.4981, 46.0424) -> (136.2073, 49.7313) centre (0, 0) ccw
  spline S148 degree 3 poles (1.9541, -144.989) (3.4732, -141.5905) (4.3732, -138.749) (4.9034, -136.5635) knots 0 0 0 0 1 1 1 1
  arc A145 (-5.4262, -133.9625) -> (-5.8041, -133.6242) centre (-5.8214, -134.0238) ccw
  arc A146 (124.2087, 49.6116) -> (122.9095, 52.7481) centre (0, 0) ccw
  spline S149 degree 3 poles (123.0504, 53.2353) (123.6498, 53.6475) (124.3604, 54.1733) (125.167, 54.8349) knots 0 0 0 0 1 1 1 1
  arc A147 (133.9625, -5.4262) -> (133.6242, -5.8041) centre (134.0238, -5.8214) ccw
  spline S150 degree 3 poles (-79.2819, 108.1193) (-79.8171, 108.6119) (-80.4878, 109.1877) (-81.3123, 109.8269) knots 0 0 0 0 1 1 1 1
  spline S151 degree 3 poles (-35.1687, -132.0485) (-35.1381, -134.2971) (-34.893, -137.2676) (-34.1682, -140.919) knots 0 0 0 0 1 1 1 1
  spline S152 degree 3 poles (-25.6078, -134.2307) (-25.1423, -133.2971) (-24.7878, -132.4873) (-24.5193, -131.8112) knots 0 0 0 0 1 1 1 1
  spline S153 degree 3 poles (-14.2918, -144.2961) (-12.4017, -141.0891) (-11.1893, -138.3662) (-10.4177, -136.2538) knots 0 0 0 0 1 1 1 1
  arc A148 (-24.0756, -131.5655) -> (-20.7287, -132.1341) centre (0, 0) ccw
  arc A149 (133.7277, 9.607) -> (133.4338, 9.1936) centre (133.8329, 9.2211) ccw
  arc A150 (144.2961, 14.2918) -> (143.8585, 18.1754) centre (0, 0) ccw
  spline S154 degree 3 poles (130.5195, 40.4758) (132.4072, 41.6981) (134.792, 43.4861) (137.4981, 46.0424) knots 0 0 0 0 1 1 1 1
  arc A151 (123.0504, 53.2353) -> (122.9095, 52.7481) centre (123.2771, 52.9058) ccw
  spline S155 degree 3 poles (143.8585, 18.1754) (140.3113, 19.3045) (137.3869, 19.8806) (135.1558, 20.1628) knots 0 0 0 0 1 1 1 1
  arc A152 (128.9824, 35.3927) -> (128.0426, 38.6549) centre (0, 0) ccw
  spline S156 degree 3 poles (-5.4262, -133.9625) (-5.3149, -134.6814) (-5.1495, -135.5497) (-4.9034, -136.5635) knots 0 0 0 0 1 1 1 1
  arc A153 (133.6242, 5.8041) -> (133.4338, 9.1936) centre (0, 0) ccw
  arc A154 (124.2087, 49.6116) -> (124.6528, 49.3667) centre (124.5801, 49.76) ccw
  arc A155 (-1.9541, -144.989) -> (1.9541, -144.989) centre (0, 0) ccw
  spline S157 degree 3 poles (125.167, 54.8349) (126.906, 56.2608) (129.0756, 58.3046) (131.4784, 61.1478) knots 0 0 0 0 1 1 1 1
  arc A156 (117.8729, 63.2067) -> (116.2308, 66.1779) centre (0, 0) ccw
  arc A157 (117.8729, 63.2067) -> (118.3417, 63.013) centre (118.2255, 63.3957) ccw
  arc A158 (116.3162, 66.6779) -> (116.2308, 66.1779) centre (116.5784, 66.3758) ccw
  spline S158 degree 3 poles (129.7827, 64.6689) (126.0616, 64.5631) (123.1111, 64.141) (120.912, 63.6705) knots 0 0 0 0 1 1 1 1
  spline S159 degree 3 poles (-10.4177, -136.2538) (-10.0596, -135.274) (-9.798, -134.4296) (-9.607, -133.7277) knots 0 0 0 0 1 1 1 1
  arc A159 (5.8041, -133.6242) -> (5.4262, -133.9625) centre (5.8214, -134.0238) ccw
  arc A160 (-20.3911, -132.5126) -> (-20.7287, -132.1341) centre (-20.7907, -132.5293) ccw
  spline S160 degree 3 poles (10.4177, -136.2538) (11.1893, -138.3662) (12.4017, -141.0891) (14.2918, -144.2961) knots 0 0 0 0 1 1 1 1
  arc A161 (128.2371, 39.1233) -> (128.0426, 38.6549) centre (128.4255, 38.7705) ccw
  spline S161 degree 3 poles (136.2073, 49.7313) (132.4978, 50.0427) (129.5185, 49.9537) (127.2805, 49.7323) knots 0 0 0 0 1 1 1 1
  arc A162 (-9.1936, -133.4338) -> (-9.607, -133.7277) centre (-9.2211, -133.8329) ccw
  spline S162 degree 3 poles (-4.9034, -136.5635) (-4.3732, -138.749) (-3.4732, -141.5905) (-1.9541, -144.989) knots 0 0 0 0 1 1 1 1
  arc A163 (9.607, -133.7277) -> (9.1936, -133.4338) centre (9.2211, -133.8329) ccw
  spline S163 degree 3 poles (49.3667, 124.6528) (49.4991, 125.3681) (49.6298, 126.2424) (49.7323, 127.2805) knots 0 0 0 0 1 1 1 1
  spline S164 degree 3 poles (103.7124, 88.9796) (102.7664, 88.5399) (101.9843, 88.1278) (101.3529, 87.7666) knots 0 0 0 0 1 1 1 1
  arc A164 (87.7666, 101.3529) -> (87.8511, 100.8528) centre (88.1139, 101.1544) ccw
  arc A165 (49.7313, 136.2073) -> (46.0424, 137.4981) centre (0, 0) ccw
  arc A166 (35.0996, 129.3963) -> (35.3927, 128.9824) centre (35.4986, 129.3682) ccw
  spline S165 degree 3 poles (46.0424, 137.4981) (43.4861, 134.792) (41.6981, 132.4072) (40.4758, 130.5195) knots 0 0 0 0 1 1 1 1
  arc A167 (52.7481, 122.9095) -> (53.2353, 123.0504) centre (52.9058, 123.2771) ccw
  spline S166 degree 3 poles (30.358, 141.7886) (28.1207, 138.8134) (26.611, 136.2434) (25.6078, 134.2307) knots 0 0 0 0 1 1 1 1
  arc A168 (90.3825, 98.5907) -> (87.8511, 100.8528) centre (0, 0) ccw
  spline S167 degree 3 poles (113.0228, 76.808) (112.0336, 76.477) (111.2103, 76.1551) (110.5424, 75.8668) knots 0 0 0 0 1 1 1 1
  arc A169 (78.7755, 108.0904) -> (76.0068, 110.0549) centre (0, 0) ccw
  arc A170 (63.013, 118.3417) -> (63.2067, 117.8729) centre (63.3957, 118.2255) ccw
  spline S168 degree 3 poles (75.4842, 123.8053) (72.3898, 121.7359) (70.116, 119.8088) (68.5043, 118.2404) knots 0 0 0 0 1 1 1 1
  arc A171 (24.0756, 131.5655) -> (24.5193, 131.8112) centre (24.1476, 131.9589) ccw
  arc A172 (91.9269, 112.1386) -> (88.8714, 114.5753) centre (0, 0) ccw
  arc A173 (108.1193, 79.2819) -> (108.0904, 78.7755) centre (108.4136, 79.0111) ccw
  spline S169 degree 3 poles (35.1687, 132.0485) (35.1381, 134.2971) (34.893, 137.2676) (34.1682, 140.919) knots 0 0 0 0 1 1 1 1
  spline S170 degree 3 poles (81.3123, 109.8269) (80.4878, 109.1877) (79.8171, 108.6119) (79.2819, 108.1193) knots 0 0 0 0 1 1 1 1
  spline S171 degree 3 poles (35.0996, 129.3963) (35.1511, 130.122) (35.183, 131.0054) (35.1687, 132.0485) knots 0 0 0 0 1 1 1 1
  arc A174 (110.0549, 76.0068) -> (108.0904, 78.7755) centre (0, 0) ccw
  arc A175 (34.1682, 140.919) -> (30.358, 141.7886) centre (0, 0) ccw
  spline S172 degree 3 poles (87.7666, 101.3529) (88.1278, 101.9843) (88.5399, 102.7664) (88.9796, 103.7124) knots 0 0 0 0 1 1 1 1
  arc A176 (78.7755, 108.0904) -> (79.2819, 108.1193) centre (79.0111, 108.4136) ccw
  arc A177 (75.8668, 110.5424) -> (76.0068, 110.0549) centre (76.2341, 110.384) ccw
  arc A178 (100.8528, 87.8511) -> (101.3529, 87.7666) centre (101.1544, 88.1139) ccw
  spline S173 degree 3 poles (76.808, 113.0228) (77.5218, 115.1555) (78.2715, 118.0402) (78.7934, 121.726) knots 0 0 0 0 1 1 1 1
  arc A179 (66.1779, 116.2308) -> (66.6779, 116.3162) centre (66.3758, 116.5784) ccw
  spline S174 degree 3 poles (63.013, 118.3417) (63.2246, 119.0377) (63.4524, 119.8918) (63.6705, 120.912) knots 0 0 0 0 1 1 1 1
  arc A180 (38.6549, 128.0426) -> (35.3927, 128.9824) centre (0, 0) ccw
  arc A181 (103.9044, 101.1409) -> (101.1409, 103.9044) centre (0, 0) ccw
  spline S175 degree 3 poles (98.5627, 90.8889) (98.9923, 91.4759) (99.4894, 92.2069) (100.0322, 93.0977) knots 0 0 0 0 1 1 1 1
  spline S176 degree 3 poles (101.1409, 103.9044) (97.6637, 102.5755) (95.018, 101.2027) (93.0977, 100.0322) knots 0 0 0 0 1 1 1 1
  spline S177 degree 3 poles (61.1478, 131.4784) (58.3046, 129.0756) (56.2608, 126.906) (54.8349, 125.167) knots 0 0 0 0 1 1 1 1
  arc A182 (131.4784, 61.1478) -> (129.7827, 64.6689) centre (0, 0) ccw
  spline S178 degree 3 poles (120.912, 63.6705) (119.8918, 63.4524) (119.0377, 63.2246) (118.3417, 63.013) knots 0 0 0 0 1 1 1 1
  arc A183 (78.7934, 121.726) -> (75.4842, 123.8053) centre (0, 0) ccw
  spline S179 degree 3 poles (54.8349, 125.167) (54.1733, 124.3604) (53.6475, 123.6498) (53.2353, 123.0504) knots 0 0 0 0 1 1 1 1
  spline S180 degree 3 poles (109.8269, 81.3123) (111.205, 83.0895) (112.8654, 85.5648) (114.5753, 88.8714) knots 0 0 0 0 1 1 1 1
  arc A184 (100.8528, 87.8511) -> (98.5907, 90.3825) centre (0, 0) ccw
  arc A185 (52.7481, 122.9095) -> (49.6116, 124.2087) centre (0, 0) ccw
  spline S181 degree 3 poles (49.7323, 127.2805) (49.9537, 129.5185) (50.0427, 132.4978) (49.7313, 136.2073) knots 0 0 0 0 1 1 1 1
  spline S182 degree 3 poles (116.3162, 66.6779) (116.8657, 67.1545) (117.5129, 67.7566) (118.2404, 68.5043) knots 0 0 0 0 1 1 1 1
  spline S183 degree 3 poles (121.726, 78.7934) (118.0402, 78.2715) (115.1555, 77.5218) (113.0228, 76.808) knots 0 0 0 0 1 1 1 1
  spline S184 degree 3 poles (118.2404, 68.5043) (119.8088, 70.116) (121.7359, 72.3898) (123.8053, 75.4842) knots 0 0 0 0 1 1 1 1
  spline S185 degree 3 poles (112.1386, 91.9269) (108.5344, 90.9957) (105.7517, 89.9277) (103.7124, 88.9796) knots 0 0 0 0 1 1 1 1
  spline S186 degree 3 poles (88.8714, 114.5753) (85.5648, 112.8654) (83.0895, 111.205) (81.3123, 109.8269) knots 0 0 0 0 1 1 1 1
  spline S187 degree 3 poles (68.5043, 118.2404) (67.7566, 117.5129) (67.1545, 116.8657) (66.6779, 116.3162) knots 0 0 0 0 1 1 1 1
  spline S188 degree 3 poles (63.6705, 120.912) (64.141, 123.1111) (64.5631, 126.0616) (64.6689, 129.7827) knots 0 0 0 0 1 1 1 1
  arc A186 (38.6549, 128.0426) -> (39.1233, 128.2371) centre (38.7705, 128.4255) ccw
  spline S189 degree 3 poles (108.1193, 79.2819) (108.6119, 79.8171) (109.1877, 80.4878) (109.8269, 81.3123) knots 0 0 0 0 1 1 1 1
  arc A187 (123.8053, 75.4842) -> (121.726, 78.7934) centre (0, 0) ccw
  arc A188 (90.3825, 98.5907) -> (90.8889, 98.5627) centre (90.6528, 98.8855) ccw
  arc A189 (110.0549, 76.0068) -> (110.5424, 75.8668) centre (110.384, 76.2341) ccw
  arc A190 (49.3667, 124.6528) -> (49.6116, 124.2087) centre (49.76, 124.5801) ccw
  spline S190 degree 3 poles (40.4758, 130.5195) (39.9087, 129.6439) (39.4658, 128.8789) (39.1233, 128.2371) knots 0 0 0 0 1 1 1 1
  arc A191 (24.0756, 131.5655) -> (20.7287, 132.1341) centre (0, 0) ccw
  spline S191 degree 3 poles (88.9796, 103.7124) (89.9277, 105.7517) (90.9957, 108.5344) (91.9269, 112.1386) knots 0 0 0 0 1 1 1 1
  spline S192 degree 3 poles (93.0977, 100.0322) (92.2069, 99.4894) (91.4759, 98.9923) (90.8889, 98.5627) knots 0 0 0 0 1 1 1 1
  spline S193 degree 3 poles (75.8668, 110.5424) (76.1551, 111.2103) (76.477, 112.0336) (76.808, 113.0228) knots 0 0 0 0 1 1 1 1
  arc A192 (98.5627, 90.8889) -> (98.5907, 90.3825) centre (98.8855, 90.6528) ccw
  spline S194 degree 3 poles (100.0322, 93.0977) (101.2027, 95.018) (102.5755, 97.6637) (103.9044, 101.1409) knots 0 0 0 0 1 1 1 1
  arc A193 (114.5753, 88.8714) -> (112.1386, 91.9269) centre (0, 0) ccw
  arc A194 (64.6689, 129.7827) -> (61.1478, 131.4784) centre (0, 0) ccw
  arc A195 (66.1779, 116.2308) -> (63.2067, 117.8729) centre (0, 0) ccw
  spline S195 degree 3 poles (-35.1687, 132.0485) (-35.183, 131.0054) (-35.1511, 130.122) (-35.0996, 129.3963) knots 0 0 0 0 1 1 1 1
  spline S196 degree 3 poles (-24.5193, 131.8112) (-24.7878, 132.4873) (-25.1423, 133.2971) (-25.6078, 134.2307) knots 0 0 0 0 1 1 1 1
  spline S197 degree 3 poles (-20.1628, 135.1558) (-20.2939, 134.1209) (-20.361, 133.2394) (-20.3911, 132.5126) knots 0 0 0 0 1 1 1 1
  spline S198 degree 3 poles (-40.4758, 130.5195) (-41.6981, 132.4072) (-43.4861, 134.792) (-46.0424, 137.4981) knots 0 0 0 0 1 1 1 1
  arc A196 (-53.2353, 123.0504) -> (-52.7481, 122.9095) centre (-52.9058, 123.2771) ccw
  arc A197 (-14.2918, 144.2961) -> (-18.1754, 143.8585) centre (0, 0) ccw
  spline S199 degree 3 poles (25.6078, 134.2307) (25.1423, 133.2971) (24.7878, 132.4873) (24.5193, 131.8112) knots 0 0 0 0 1 1 1 1
  spline S200 degree 3 poles (-49.7323, 127.2805) (-49.6298, 126.2424) (-49.4991, 125.3681) (-49.3667, 124.6528) knots 0 0 0 0 1 1 1 1
  spline S201 degree 3 poles (20.1628, 135.1558) (19.8806, 137.3869) (19.3045, 140.3113) (18.1754, 143.8585) knots 0 0 0 0 1 1 1 1
  spline S202 degree 3 poles (5.4262, 133.9625) (5.3149, 134.6814) (5.1495, 135.5497) (4.9034, 136.5635) knots 0 0 0 0 1 1 1 1
  arc A198 (-63.2067, 117.8729) -> (-63.013, 118.3417) centre (-63.3957, 118.2255) ccw
  spline S203 degree 3 poles (-66.6779, 116.3162) (-67.1545, 116.8657) (-67.7566, 117.5129) (-68.5043, 118.2404) knots 0 0 0 0 1 1 1 1
  spline S204 degree 3 poles (-78.7934, 121.726) (-78.2715, 118.0402) (-77.5218, 115.1555) (-76.808, 113.0228) knots 0 0 0 0 1 1 1 1
  arc A199 (9.1936, 133.4338) -> (5.8041, 133.6242) centre (0, 0) ccw
  arc A200 (-49.6116, 124.2087) -> (-49.3667, 124.6528) centre (-49.76, 124.5801) ccw
  arc A201 (-24.5193, 131.8112) -> (-24.0756, 131.5655) centre (-24.1476, 131.9589) ccw
  arc A202 (-76.0068, 110.0549) -> (-78.7755, 108.0904) centre (0, 0) ccw
  spline S205 degree 3 poles (-49.7313, 136.2073) (-50.0427, 132.4978) (-49.9537, 129.5185) (-49.7323, 127.2805) knots 0 0 0 0 1 1 1 1
  arc A203 (-49.6116, 124.2087) -> (-52.7481, 122.9095) centre (0, 0) ccw
  arc A204 (-63.2067, 117.8729) -> (-66.1779, 116.2308) centre (0, 0) ccw
  spline S206 degree 3 poles (-53.2353, 123.0504) (-53.6475, 123.6498) (-54.1733, 124.3604) (-54.8349, 125.167) knots 0 0 0 0 1 1 1 1
  arc A205 (-66.6779, 116.3162) -> (-66.1779, 116.2308) centre (-66.3758, 116.5784) ccw
  arc A206 (-9.607, 133.7277) -> (-9.1936, 133.4338) centre (-9.2211, 133.8329) ccw
  arc A207 (-79.2819, 108.1193) -> (-78.7755, 108.0904) centre (-79.0111, 108.4136) ccw
  spline S207 degree 3 poles (-9.607, 133.7277) (-9.798, 134.4296) (-10.0596, 135.274) (-10.4177, 136.2538) knots 0 0 0 0 1 1 1 1
  arc A208 (-61.1478, 131.4784) -> (-64.6689, 129.7827) centre (0, 0) ccw
  spline S208 degree 3 poles (-39.1233, 128.2371) (-39.4658, 128.8789) (-39.9087, 129.6439) (-40.4758, 130.5195) knots 0 0 0 0 1 1 1 1
  arc A209 (5.4262, 133.9625) -> (5.8041, 133.6242) centre (5.8214, 134.0238) ccw
  spline S209 degree 3 poles (14.2918, 144.2961) (12.4017, 141.0891) (11.1893, 138.3662) (10.4177, 136.2538) knots 0 0 0 0 1 1 1 1
  spline S210 degree 3 poles (4.9034, 136.5635) (4.3732, 138.749) (3.4732, 141.5905) (1.9541, 144.989) knots 0 0 0 0 1 1 1 1
  arc A210 (20.3911, 132.5126) -> (20.7287, 132.1341) centre (20.7907, 132.5293) ccw
  arc A211 (-35.3927, 128.9824) -> (-38.6549, 128.0426) centre (0, 0) ccw
  arc A212 (-20.7287, 132.1341) -> (-24.0756, 131.5655) centre (0, 0) ccw
  arc A213 (-35.3927, 128.9824) -> (-35.0996, 129.3963) centre (-35.4986, 129.3682) ccw
  arc A214 (18.1754, 143.8585) -> (14.2918, 144.2961) centre (0, 0) ccw
  spline S211 degree 3 poles (10.4177, 136.2538) (10.0596, 135.274) (9.798, 134.4296) (9.607, 133.7277) knots 0 0 0 0 1 1 1 1
  spline S212 degree 3 poles (-10.4177, 136.2538) (-11.1893, 138.3662) (-12.4017, 141.0891) (-14.2918, 144.2961) knots 0 0 0 0 1 1 1 1
  spline S213 degree 3 poles (-64.6689, 129.7827) (-64.5631, 126.0616) (-64.141, 123.1111) (-63.6705, 120.912) knots 0 0 0 0 1 1 1 1
  arc A215 (-5.8041, 133.6242) -> (-5.4262, 133.9625) centre (-5.8214, 134.0238) ccw
  arc A216 (-30.358, 141.7886) -> (-34.1682, 140.919) centre (0, 0) ccw
  spline S214 degree 3 poles (20.3911, 132.5126) (20.361, 133.2394) (20.2939, 134.1209) (20.1628, 135.1558) knots 0 0 0 0 1 1 1 1
  arc A217 (-20.7287, 132.1341) -> (-20.3911, 132.5126) centre (-20.7907, 132.5293) ccw
  spline S215 degree 3 poles (-34.1682, 140.919) (-34.893, 137.2676) (-35.1381, 134.2971) (-35.1687, 132.0485) knots 0 0 0 0 1 1 1 1
  arc A218 (-39.1233, 128.2371) -> (-38.6549, 128.0426) centre (-38.7705, 128.4255) ccw
  spline S216 degree 3 poles (-63.6705, 120.912) (-63.4524, 119.8918) (-63.2246, 119.0377) (-63.013, 118.3417) knots 0 0 0 0 1 1 1 1
  arc A219 (-75.4842, 123.8053) -> (-78.7934, 121.726) centre (0, 0) ccw
  spline S217 degree 3 poles (-54.8349, 125.167) (-56.2608, 126.906) (-58.3046, 129.0756) (-61.1478, 131.4784) knots 0 0 0 0 1 1 1 1
  spline S218 degree 3 poles (-68.5043, 118.2404) (-70.116, 119.8088) (-72.3898, 121.7359) (-75.4842, 123.8053) knots 0 0 0 0 1 1 1 1
  spline S219 degree 3 poles (-76.808, 113.0228) (-76.477, 112.0336) (-76.1551, 111.2103) (-75.8668, 110.5424) knots 0 0 0 0 1 1 1 1
  spline S220 degree 3 poles (-25.6078, 134.2307) (-26.611, 136.2434) (-28.1207, 138.8134) (-30.358, 141.7886) knots 0 0 0 0 1 1 1 1
  arc A220 (-76.0068, 110.0549) -> (-75.8668, 110.5424) centre (-76.2341, 110.384) ccw
  arc A221 (-5.8041, 133.6242) -> (-9.1936, 133.4338) centre (0, 0) ccw
  spline S221 degree 3 poles (-18.1754, 143.8585) (-19.3045, 140.3113) (-19.8806, 137.3869) (-20.1628, 135.1558) knots 0 0 0 0 1 1 1 1
  arc A222 (9.1936, 133.4338) -> (9.607, 133.7277) centre (9.2211, 133.8329) ccw
  arc A223 (-46.0424, 137.4981) -> (-49.7313, 136.2073) centre (0, 0) ccw
  arc A224 (1.9541, 144.989) -> (-1.9541, 144.989) centre (0, 0) ccw
  spline S222 degree 3 poles (-4.9034, 136.5635) (-5.1495, 135.5497) (-5.3149, 134.6814) (-5.4262, 133.9625) knots 0 0 0 0 1 1 1 1
  spline S223 degree 3 poles (-1.9541, 144.989) (-3.4732, 141.5905) (-4.3732, 138.749) (-4.9034, 136.5635) knots 0 0 0 0 1 1 1 1
extrude "Extrude1" add sketch "sketch 243" along normal blind 8 makes body 1 in component "Spur Gear (56 teeth)"
sketch "Sketch1" plane through (0, 0, 0) normal (0, 1, 0) x (1, 0, 0) in component "Spur Gear (56 teeth)"
  circle A0 centre (0, 0) radius 140 construction